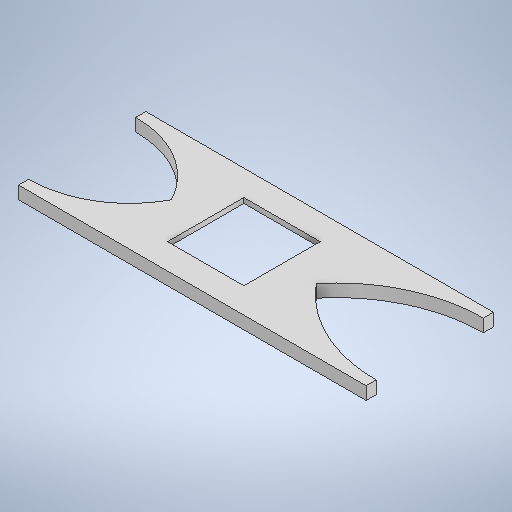
# Autodesk Inventor part: Spin Arrest
Saved by Autodesk Inventor 2025 (Build 290162000, 162)
## iProperties
Created: 2024-11-04
Part Number: Spin Arrest
Material: Generic
Document SubType Name: Modeling
Designer: Caleb Fangmeier
Density: 1 g/cm^3
Appearance: Default
Author: Caleb Fangmeier
Autodesk Inventor part; units mm, degrees
ref_plane "YZ Plane" through (0, 0, 0) normal (1, 0, 0) x (0, 1, 0)
ref_plane "XZ Plane" through (0, 0, 0) normal (0, 1, 0) x (-1, 0, 0)
ref_plane "XY Plane" through (0, 0, 0) normal (0, 0, 1) x (1, 0, 0)
sketch "Sketch1" plane through (0, 0, 0) normal (0, 1, 0) x (-1, 0, 0)
  line L0 (-68.2625, -25) -> (68.2625, -25)
  line L1 (68.2625, -25) -> (68.2625, 25)
  line L2 (68.2625, 25) -> (-68.2625, 25)
  line L3 (-68.2625, 25) -> (-68.2625, -25)
  line L4 (-68.2625, -25) -> (68.2625, 25) construction
  line L5 (68.2625, -25) -> (-68.2625, 25) construction
  point P0 (0, 0)
  dimension "d0" = 136.525
  dimension "d1" = 50
  constraints: 12 end point, 2 midpoint, 2 parallel, 1 horizontal, 1 perpendicular
  measures "d0" distance of L1.end L2.end
  measures "d1" distance of L0.end L1.end
extrude "Extrusion1" add sketch "Sketch1" along normal blind 5
sketch "Sketch2" plane through (0, 0, 0) normal (0, -1, 0) x (1, 0, 0)
  circle A0 centre (-4.7625, 0) radius 25.5
  line L0 (-68.2625, -25) -> (-68.2625, 25) projected
  line L1 (-20.5818, -20) -> (11.0568, -20)
  line L2 (-20.5818, 20) -> (11.0568, 20)
  point P0 (0, 0)
  dimension "d4" = 51
  dimension "d5" = 63.5
  dimension "d6" = 40
  dimension "d7" = 20
  constraints: 4 end point, 4 point on circle, 1 centre point, 1 horizontal, 1 horizontal alignment, 1 parallel
  measures "d4" diameter of A0
  measures "d5" distance from line of L0 A0.centre
  measures "d6" distance between parallel lines of L1 L2
  measures "d7" distance from line of L1 point (0, 0)
extrude "Extrusion2" cut sketch "Sketch2" against normal blind 3 contours A0 L1 L2
sketch "Sketch3" plane through (0, 0, 0) normal (0, -1, 0) x (1, 0, 0)
  line L0 (68.2625, 25) -> (68.2625, -25) projected
  arc A0 (23.7375, 0) -> (68.2625, -21) centre (68.2625, 36.7018) ccw
  arc A1 (68.2625, 21) -> (23.7375, 0) centre (68.2625, -36.7018) ccw
  arc A2 (11.0568, -20) -> (11.0568, 20) centre (-4.7625, 0) ccw projected
  line L1 (-68.2625, -25) -> (-68.2625, 25) projected
  arc A3 (-68.2625, -21) -> (-33.2625, 0) centre (-68.2625, 18.6667) ccw
  arc A4 (-33.2625, 0) -> (-68.2625, 21) centre (-68.2625, -18.6667) ccw
  arc A5 (-20.5818, 20) -> (-20.5818, -20) centre (-4.7625, 0) ccw projected
  line L2 (10.2375, 15) -> (-19.7625, 15)
  line L3 (-19.7625, 15) -> (-19.7625, -15)
  line L4 (-19.7625, -15) -> (10.2375, -15)
  line L5 (10.2375, -15) -> (10.2375, 15)
  line L6 (10.2375, 15) -> (-19.7625, -15) construction
  line L7 (-19.7625, 15) -> (10.2375, -15) construction
  point P0 (0, 0)
  point P1 (20.7375, 0)
  point P2 (-30.2625, 0)
  dimension "d10" = 4
  dimension "d11" = 4
  dimension "d12" = 3
  dimension "d13" = 4
  dimension "d14" = 4
  dimension "d15" = 3
  dimension "d16" = 30
  dimension "d17" = 30
  constraints: 12 end point, 10 point on circle, 4 centre point, 4 point on line, 2 equal radius, 2 horizontal alignment, 2 line through centre, 2 midpoint, 2 parallel, 1 horizontal, 1 perpendicular
  measures "d10" distance of L0.end A0.end
  measures "d11" distance of L0.start A1.start
  measures "d12" distance of point (20.737, 0) A0.start
  measures "d13" distance of L1.start A3.start
  measures "d14" distance of L1.end A4.end
  measures "d15" distance of A3.end point (-30.262, 0)
  measures "d16" distance of L4.end L3.end
  measures "d17" distance of L3.end L2.end
extrude "Extrusion3" cut sketch "Sketch3" against normal through all
equation "\"d7\" = 0.5 * d6"
equation "\"d11\" = d10"
equation "\"d14\" = d13"
body "Solid1"
